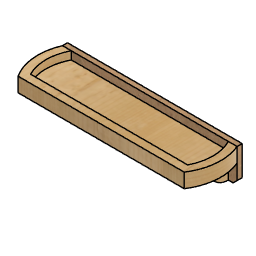
model (Autodesk Fusion 360 design; units mm, degrees)
Autodesk Fusion 360 part; units mm, degrees
sketch "Sketch1" plane through (0, 0, 0) normal (0, 0, 1) x (1, 0, 0)
  line L0 (0, 0) -> (197, 0)
  arc A0 (197, 0) -> (197, 51) centre (148.105, 25.5) ccw
  line L1 (197, 51) -> (0, 51)
  arc A1 (0, 51) -> (0, 0) centre (48.895, 25.5) ccw
  line L2 (197, 51) -> (197, 0) construction
  line L3 (0, 0) -> (0, 51) construction
  line L4 (-6.25, 25.5) -> (203.25, 25.5) construction
  line L5 (98.5, 51) -> (98.5, 0) construction
  line L6 (-5.7275, -10) -> (202.7275, -10)
  arc A2 (202.7275, -10) -> (208.0518, 51) centre (148.105, 25.5) ccw
  arc A3 (-11.0518, 51) -> (-5.7275, -10) centre (48.895, 25.5) ccw
  line L7 (-11.0518, 51) -> (0, 51)
  line L8 (197, 51) -> (208.0518, 51)
  point P0 (-6.25, 25.5)
  point P1 (203.25, 25.5)
  dimension "d255" = 51
  dimension "d256" = 197
  dimension "d257" = 209.5
  dimension "d258" = 10
  constraint coincident L0.start A1.end
  constraint horizontal L0
  constraint parallel L0 L1
  constraint vertical L3
  constraint vertical L2
  constraint midpoint A1 P0
  constraint midpoint A0 P1
  constraint coincident P0 L4.start
  constraint coincident P1 L4.end
  constraint midpoint L1 L5.start
  constraint midpoint L0 L5.end
  constraint midpoint L4 L5
  constraint horizontal L8
  constraint horizontal L7
  measures "d255" vertical distance of L0.end A0.end
  measures "d256" distance of L0.start L0.end
  measures "d257" distance of P0 P1
extrude "Extrude1" add sketch "Sketch1" along normal blind 8 contours L0 A0 L1 A1 makes body 1
extrude "Extrude2" add sketch "Sketch1" along normal blind 18 contours L0 A0 A1 L6 A2 A3 L7 L8 bodies 1
sketch "Sketch2" plane through (0, 0, 0) normal (1, 0, 0) x (0, 1, 0)
  line L0 (51, 0) -> (27, 0)
  line L1 (51, 0) -> (51, -24)
  arc A0 (27, 0) -> (51, -24) centre (51, 0) ccw
  line L2 (51, -24) -> (57.35, -24)
  line L3 (57.35, -24) -> (57.35, 18)
  line L4 (57.35, 18) -> (51, 18)
  line L5 (51, 18) -> (51, -24)
  point P0 (51, 0)
  point P1 (-10, 0)
  point P2 (51, 18)
  dimension "d263" = 24
  dimension "d264" = 6.35
  constraint coincident P0 L0.start
  constraint horizontal L0
  constraint vertical L1
  constraint horizontal L2
  constraint vertical L3
  constraint horizontal L4
  constraint vertical L5
  constraint coincident P2 L4.end
  measures "d263" vertical distance of P0 L1.end
  measures "d264" distance of L3.end P2
extrude "Extrude3" add sketch "Sketch2" along normal up to surface (219.1036 mm away) from surface at -11.0518 separate body contours L1 L2 L3 L4 L5 makes body 2
extrude "Extrude4" add sketch "Sketch2" along normal blind 18 separate body contours L0 L1 A0 L5 makes body 3
ref_plane "WorkPlane1" through (98.5, 54.175, -3) normal (1, 0, 0) x (0, 0, -1)
mirror "Mirror1" about plane through (98.5, 54.175, -3) normal (1, 0, 0) of bodies 3 makes body 4
chamfer "Chamfer1" distance 5 angle 45 2 edges at (-11.0518, 54.175, -24) (208.0518, 54.175, -24) on bodies 2
equation "outerWidth = 49.4 mm"
equation "innerWidth = 41.5 mm"
equation "baseThickness = 4.8 mm"
equation "arcDepth = 5.5 mm"
equation "totalLength = 260 mm"
equation "frontHumpOffset = 54 mm"
equation "humpLength = 50 mm"
equation "humpHeight = 45 mm"
equation "knobFrontInset = 4.3 mm"
equation "mountThickness = 5 mm"
equation "screwOD = 10 mm"
equation "screwID = 4.5 mm"
equation "screwChamfer = 4 mm"
equation "toteExtension = 18 mm"
equation "toteExtensionWidth = 26 mm"
equation "knobDiameter = 26.3 mm"
equation "d264 = 1/4\""
